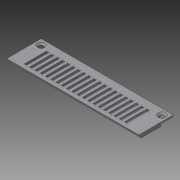
# Autodesk Inventor part: back cover
Saved by Autodesk Inventor 2015 (Build 190159000, 159)
## iProperties
Created: 2019-01-20
Part Number: back cover
Material: Generic
Document SubType Name: Modeling
Designer: Toby
Density: 1 g/cm^3
Appearance: Default
Author: Toby
Autodesk Inventor part; units mm, degrees
ref_plane "YZ Plane" through (0, 0, 0) normal (1, 0, 0) x (0, 1, 0)
ref_plane "XZ Plane" through (0, 0, 0) normal (0, 1, 0) x (-1, 0, 0)
ref_plane "XY Plane" through (0, 0, 0) normal (0, 0, 1) x (1, 0, 0)
sketch "Sketch1" plane through (0, 0, 0) normal (0, 0, 1) x (1, 0, 0)
  line L0 (-58.6081, 2.801) -> (41.3919, 2.801)
  line L1 (41.3919, 2.801) -> (41.3919, -23.199)
  line L2 (41.3919, -23.199) -> (-58.6081, -23.199)
  line L3 (-58.6081, -23.199) -> (-58.6081, 2.801)
  point P0 (0, 0)
  dimension "d0" = 100
  dimension "d1" = 26
  constraints: 8 end point, 2 parallel, 1 horizontal, 1 perpendicular
  measures "d0" distance of L0.start L0.end
  measures "d1" distance between parallel lines of L2 L0
extrude "Extrusion1" add sketch "Sketch1" along normal blind 1.2
sketch "Sketch2" plane through (0, 0, 1.2) normal (0, 0, 1) x (1, 0, 0)
  line L0 (41.3919, 2.801) -> (-58.6081, 2.801) projected
  line L1 (-58.6081, 2.801) -> (-58.6081, -23.199) projected
  line L2 (41.3919, -23.199) -> (41.3919, 2.801) projected
  point P0 (0, 0)
  point P1 (-54.4081, -1.399)
  point P2 (37.1919, -1.399)
  dimension "d4" = 4.2
  dimension "d5" = 4.2
  dimension "d6" = 4.2
  dimension "d7" = 4.2
  measures "d4" distance from line of L0 point (-54.408, -1.399)
  measures "d5" distance from line of L0 point (37.192, -1.399)
  measures "d6" distance from line of L1 point (-54.408, -1.399)
  measures "d7" distance from line of L2 point (37.192, -1.399)
hole "Hole1" at (-54.4081, -1.399, 1.2) at (37.1919, -1.399, 1.2) direction (0, 0, -1) diameter 3 depth 8 tip angle 118 countersink diameter 6 countersink angle 90
sketch "Sketch3" plane through (0, 0, 0) normal (0, 0, -1) x (-1, 0, 0)
  line L0 (-33.3919, 1.601) -> (50.6081, 1.601)
  line L1 (50.6081, 1.601) -> (50.6081, -0.799)
  line L2 (50.6081, -0.799) -> (-33.3919, -0.799)
  line L3 (-33.3919, -0.799) -> (-33.3919, 1.601)
  line L4 (-41.3919, 2.801) -> (58.6081, 2.801) projected
  line L5 (-41.3919, 2.801) -> (-41.3919, -23.199) projected
  line L6 (58.6081, -23.199) -> (58.6081, 2.801) projected
  point P0 (0, 0)
  dimension "d15" = 1.2
  dimension "d16" = 8
  dimension "d17" = 8
  dimension "d18" = 2.4
  constraints: 8 end point, 2 parallel, 1 horizontal, 1 perpendicular
  measures "d15" distance between parallel lines of L4 L0
  measures "d16" distance between parallel lines of L5 L3
  measures "d17" distance between parallel lines of L6 L1
  measures "d18" distance between parallel lines of L2 L0
extrude "Extrusion2" add sketch "Sketch3" along normal blind 3
sketch "Sketch4" plane through (0, 0, 0) normal (0, 0, -1) x (-1, 0, 0)
  line L0 (-40.1919, -5.199) -> (-38.1919, -5.199)
  line L1 (-38.1919, -5.199) -> (-38.1919, -20.199)
  line L2 (-38.1919, -20.199) -> (-40.1919, -20.199)
  line L3 (-40.1919, -20.199) -> (-40.1919, -5.199)
  line L4 (57.4081, -5.199) -> (55.4081, -5.199)
  line L5 (55.4081, -5.199) -> (55.4081, -20.199)
  line L6 (55.4081, -20.199) -> (57.4081, -20.199)
  line L7 (57.4081, -20.199) -> (57.4081, -5.199)
  line L8 (-41.3919, 2.801) -> (-41.3919, -23.199) projected
  line L9 (58.6081, -23.199) -> (58.6081, 2.801) projected
  line L10 (58.6081, 2.801) -> (-41.3919, 2.801) projected
  line L11 (-41.3919, -23.199) -> (58.6081, -23.199) projected
  point P0 (0, 0)
  dimension "d21" = 1.2
  dimension "d22" = 2
  dimension "d23" = 2
  dimension "d24" = 1.2
  dimension "d25" = 8
  dimension "d26" = 3
  constraints: 16 end point, 4 parallel, 2 horizontal, 2 perpendicular, 2 point on line
  measures "d21" distance between parallel lines of L8 L3
  measures "d22" distance between parallel lines of L1 L3
  measures "d23" distance between parallel lines of L7 L5
  measures "d24" distance between parallel lines of L9 L7
  measures "d25" distance between parallel lines of L10 L4
  measures "d26" distance between parallel lines of L11 L2
extrude "Extrusion3" add sketch "Sketch4" along normal blind 3 contours L0 L1 L2 L3 | L7 L6 L5 L4
sketch "Sketch5" plane through (0, 0, 1.2) normal (0, 0, 1) x (1, 0, 0)
  line L0 (-48.6081, -3.199) -> (-46.6081, -3.199)
  line L1 (-46.6081, -3.199) -> (-46.6081, -20.199)
  line L2 (-46.6081, -20.199) -> (-48.6081, -20.199)
  line L3 (-48.6081, -20.199) -> (-48.6081, -3.199)
  line L4 (-58.6081, 2.801) -> (-58.6081, -23.199) projected
  line L5 (41.3919, 2.801) -> (-58.6081, 2.801) projected
  line L6 (-58.6081, -23.199) -> (41.3919, -23.199) projected
  line L7 (-44.6081, -3.199) -> (-42.6081, -3.199)
  line L8 (-42.6081, -3.199) -> (-42.6081, -20.199)
  line L9 (-42.6081, -20.199) -> (-44.6081, -20.199)
  line L10 (-44.6081, -20.199) -> (-44.6081, -3.199)
  line L11 (-40.6081, -3.199) -> (-38.6081, -3.199)
  line L12 (-38.6081, -3.199) -> (-38.6081, -20.199)
  line L13 (-38.6081, -20.199) -> (-40.6081, -20.199)
  line L14 (-40.6081, -20.199) -> (-40.6081, -3.199)
  line L15 (-36.6081, -3.199) -> (-34.6081, -3.199)
  line L16 (-34.6081, -3.199) -> (-34.6081, -20.199)
  line L17 (-34.6081, -20.199) -> (-36.6081, -20.199)
  line L18 (-36.6081, -20.199) -> (-36.6081, -3.199)
  line L19 (-32.6081, -3.199) -> (-30.6081, -3.199)
  line L20 (-30.6081, -3.199) -> (-30.6081, -20.199)
  line L21 (-30.6081, -20.199) -> (-32.6081, -20.199)
  line L22 (-32.6081, -20.199) -> (-32.6081, -3.199)
  line L23 (-28.6081, -3.199) -> (-26.6081, -3.199)
  line L24 (-26.6081, -3.199) -> (-26.6081, -20.199)
  line L25 (-26.6081, -20.199) -> (-28.6081, -20.199)
  line L26 (-28.6081, -20.199) -> (-28.6081, -3.199)
  line L27 (-24.6081, -3.199) -> (-22.6081, -3.199)
  line L28 (-22.6081, -3.199) -> (-22.6081, -20.199)
  line L29 (-22.6081, -20.199) -> (-24.6081, -20.199)
  line L30 (-24.6081, -20.199) -> (-24.6081, -3.199)
  line L31 (-20.6081, -3.199) -> (-18.6081, -3.199)
  line L32 (-18.6081, -3.199) -> (-18.6081, -20.199)
  line L33 (-18.6081, -20.199) -> (-20.6081, -20.199)
  line L34 (-20.6081, -20.199) -> (-20.6081, -3.199)
  line L35 (-16.6081, -3.199) -> (-14.6081, -3.199)
  line L36 (-14.6081, -3.199) -> (-14.6081, -20.199)
  line L37 (-14.6081, -20.199) -> (-16.6081, -20.199)
  line L38 (-16.6081, -20.199) -> (-16.6081, -3.199)
  line L39 (-12.6081, -3.199) -> (-10.6081, -3.199)
  line L40 (-10.6081, -3.199) -> (-10.6081, -20.199)
  line L41 (-10.6081, -20.199) -> (-12.6081, -20.199)
  line L42 (-12.6081, -20.199) -> (-12.6081, -3.199)
  line L43 (-8.6081, -3.199) -> (-6.6081, -3.199)
  line L44 (-6.6081, -3.199) -> (-6.6081, -20.199)
  line L45 (-6.6081, -20.199) -> (-8.6081, -20.199)
  line L46 (-8.6081, -20.199) -> (-8.6081, -3.199)
  line L47 (-4.6081, -3.199) -> (-2.6081, -3.199)
  line L48 (-2.6081, -3.199) -> (-2.6081, -20.199)
  line L49 (-2.6081, -20.199) -> (-4.6081, -20.199)
  line L50 (-4.6081, -20.199) -> (-4.6081, -3.199)
  line L51 (-0.6081, -3.199) -> (1.3919, -3.199)
  line L52 (1.3919, -3.199) -> (1.3919, -20.199)
  line L53 (1.3919, -20.199) -> (-0.6081, -20.199)
  line L54 (-0.6081, -20.199) -> (-0.6081, -3.199)
  line L55 (3.3919, -3.199) -> (5.3919, -3.199)
  line L56 (5.3919, -3.199) -> (5.3919, -20.199)
  line L57 (5.3919, -20.199) -> (3.3919, -20.199)
  line L58 (3.3919, -20.199) -> (3.3919, -3.199)
  line L59 (7.3919, -3.199) -> (9.3919, -3.199)
  line L60 (9.3919, -3.199) -> (9.3919, -20.199)
  line L61 (9.3919, -20.199) -> (7.3919, -20.199)
  line L62 (7.3919, -20.199) -> (7.3919, -3.199)
  line L63 (11.3919, -3.199) -> (13.3919, -3.199)
  line L64 (13.3919, -3.199) -> (13.3919, -20.199)
  line L65 (13.3919, -20.199) -> (11.3919, -20.199)
  line L66 (11.3919, -20.199) -> (11.3919, -3.199)
  line L67 (15.3919, -3.199) -> (17.3919, -3.199)
  line L68 (17.3919, -3.199) -> (17.3919, -20.199)
  line L69 (17.3919, -20.199) -> (15.3919, -20.199)
  line L70 (15.3919, -20.199) -> (15.3919, -3.199)
  line L71 (19.3919, -3.199) -> (21.3919, -3.199)
  line L72 (21.3919, -3.199) -> (21.3919, -20.199)
  line L73 (21.3919, -20.199) -> (19.3919, -20.199)
  line L74 (19.3919, -20.199) -> (19.3919, -3.199)
  line L75 (23.3919, -3.199) -> (25.3919, -3.199)
  line L76 (25.3919, -3.199) -> (25.3919, -20.199)
  line L77 (25.3919, -20.199) -> (23.3919, -20.199)
  line L78 (23.3919, -20.199) -> (23.3919, -3.199)
  line L79 (27.3919, -20.199) -> (27.3919, -3.199)
  line L80 (27.3919, -3.199) -> (29.3919, -3.199)
  line L81 (29.3919, -3.199) -> (29.3919, -20.199)
  line L82 (29.3919, -20.199) -> (27.3919, -20.199)
  point P0 (0, 0)
  point P1 (-50.6081, -3.199)
  dimension "d29" = 10
  dimension "d30" = 2
  dimension "d31" = 6
  dimension "d32" = 3
  dimension "d33" = 2
  dimension "d34" = 2
  dimension "d35" = 2
  dimension "d36" = 2
  dimension "d37" = 2
  dimension "d38" = 2
  dimension "d39" = 2
  dimension "d40" = 2
  dimension "d41" = 2
  dimension "d42" = 2
  dimension "d43" = 2
  dimension "d44" = 2
  dimension "d45" = 2
  dimension "d46" = 2
  dimension "d47" = 2
  dimension "d48" = 2
  dimension "d49" = 2
  dimension "d50" = 2
  dimension "d51" = 2
  dimension "d52" = 2
  constraints: 160 end point, 40 parallel, 20 horizontal, 20 perpendicular
  measures "d29" distance between parallel lines of L4 L3
  measures "d30" distance of L0.start L0.end
  measures "d31" distance between parallel lines of L5 L0
  measures "d32" distance between parallel lines of L6 L2
  measures "d33" distance from line of L3 point (-50.608, -3.199)
  measures "d34" distance of L10.end L7.end
  measures "d35" distance of L14.end L11.end
  measures "d36" distance of L18.end L15.end
  measures "d37" distance of L22.end L19.end
  measures "d38" distance of L26.end L23.end
  measures "d39" distance of L30.end L27.end
  measures "d40" distance of L34.end L31.end
  measures "d41" distance of L38.end L35.end
  measures "d42" distance of L42.end L39.end
  measures "d43" distance of L46.end L43.end
  measures "d44" distance of L50.end L47.end
  measures "d45" distance of L54.end L51.end
  measures "d46" distance of L58.end L55.end
  measures "d47" distance of L62.end L59.end
  measures "d48" distance of L66.end L63.end
  measures "d49" distance of L70.end L67.end
  measures "d50" distance of L74.end L71.end
  measures "d51" distance of L78.end L75.end
  measures "d52" distance of L79.end L81.start
extrude "Extrusion4" cut sketch "Sketch5" against normal blind 3
body "Solid1"
